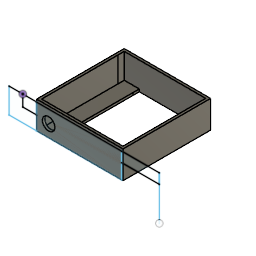
Battery_Body (Autodesk Fusion 360 design; units mm, degrees)
part number: 2026-04-07-23-47-39-558
Autodesk Fusion 360 part; units mm, degrees
sketch "Sketch1" plane through (0, 0, 0) normal (0, 1, 0) x (1, 0, 0)
  line L0 (0, 0) -> (11, 0)
  line L1 (11, 0) -> (11, 9)
  line L2 (11, 9) -> (0, 9)
  line L3 (0, 9) -> (0, 0)
  line L4 (11, 0) -> (79, 0)
  line L5 (79, 0) -> (79, 20)
  line L6 (79, 20) -> (11, 20)
  line L7 (11, 20) -> (11, 0)
  line L8 (11, 20) -> (-11, 20)
  line L9 (-11, 20) -> (-11, 0)
  line L10 (-11, 0) -> (0, 0)
  line L11 (79, 0) -> (109, 0)
  line L12 (109, 0) -> (109, 8)
  line L13 (109, 8) -> (79, 8)
  line L14 (109, 0) -> (109, 35)
  dimension "d2" = 9
  dimension "d3" = 30
  dimension "d4" = 8
  dimension "d5" = 35
  dimension "d6" = 68
  dimension "d7" = 20
  constraint coincident L0.start L3.end
  constraint horizontal L0
  constraint perpendicular L0 L1
  constraint perpendicular L1 L2
  constraint perpendicular L0 L3
  constraint perpendicular L1 L4
  constraint perpendicular L4 L5
  constraint perpendicular L5 L6
  constraint perpendicular L7 L8
  constraint perpendicular L6 L9
  constraint perpendicular L3 L10
  constraint perpendicular L5 L11
  constraint perpendicular L11 L12
  constraint coincident L5 L13.end
  constraint perpendicular L5 L13
  constraint perpendicular L11 L14
  measures "d2" distance of L0.end L1.end
  measures "d3" distance of L4.end L11.end
  measures "d4" distance of L11.end L12.end
  measures "d5" distance of L11.end L14.end
  measures "d6" distance of L5.end L6.end
  measures "d7" distance of L8.end L9.end
extrude "Extrude1" add sketch "Sketch1" along normal blind 65 contours L1 L4 L5 L6 L7
shell "Shell1" thickness 2 removed faces 1 at (33.6667, 21.6667, 0)
hole "Hole1" at (20.5975, 0, -10.3145) direction (0, 1, 0) diameter 10 depth 5 tip angle 180
sketch "Sketch2" plane through (0, 0, -18) normal (0, 0, 1) x (-1, 0, 0)
  line L0 (-13, -2) -> (-77, -2)
  line L1 (-77, -2) -> (-77, -63)
  line L2 (-77, -63) -> (-13, -63)
  line L3 (-13, -63) -> (-13, -2)
  line L4 (-13, -2) -> (-25, -2)
  line L5 (-25, -63) -> (-25, -2)
  line L6 (-77, -2) -> (-65, -2)
  line L7 (-65, -2) -> (-65, -63)
  line L8 (-77, -63) -> (-77, -2)
  line L9 (-25, -2) -> (-65, -2)
  line L10 (-65, -63) -> (-25, -63)
  dimension "d14" = 12
  constraint coincident L0.start L3.end
  constraint coincident L0 L4.end
  constraint coincident L2 L5.start
  constraint perpendicular L4 L5
  constraint coincident L0.end L1.start
  constraint perpendicular L1 L6
  constraint coincident L2 L7.end
  constraint perpendicular L2 L7
  constraint coincident L1.end L2.start
  measures "d14" distance of L0.end L6.end
extrude "Extrude2" cut sketch "Sketch2" against normal blind 5 contours L0 L2 L5 L7 L9 L10
extrude "Extrude3" add 1 faces at (34.3333, 64.3333, 0) along direction (0, 0, 1) blind 2
extrude "Extrude4" add 1 faces at (33.6667, 65, -5.3333) along direction (0, 1, 0) blind 5
sketch "Sketch3" plane through (0, 0, 2) normal (0, 0, 1) x (-1, 0, 0)
  line L0 (-13, -2) -> (-13, -63)
  line L1 (-13, -63) -> (-77, -63)
  line L2 (-77, -63) -> (-77, -2)
  line L3 (-77, -2) -> (-13, -2)
  line L4 (-11, 0) -> (-79, 0)
  line L5 (-79, 0) -> (-79, -70)
  line L6 (-79, -70) -> (-11, -70)
  line L7 (-11, -70) -> (-11, 0)
  line L8 (-77, -63) -> (-77, -68)
  line L9 (-77, -68) -> (-13, -68)
  line L10 (-13, -68) -> (-13, -63)
  constraint coincident L1.end L2.start
  constraint perpendicular L1 L8
  constraint perpendicular L8 L9
  constraint coincident L0.end L1.start
extrude "Extrude5" cut sketch "Sketch3" against normal blind 20 contours L1 L8 L9 L10
sketch "Sketch4" plane through (0, 0, -18) normal (0, 0, 1) x (-1, 0, 0)
  line L0 (-25, -2) -> (-25, -63)
  line L1 (-25, -63) -> (-65, -63)
  line L2 (-65, -63) -> (-65, -2)
  line L3 (-65, -2) -> (-77, -2)
  line L4 (-77, -2) -> (-77, -68)
  line L5 (-77, -68) -> (-13, -68)
  line L6 (-13, -68) -> (-13, -63)
  line L7 (-13, -63) -> (-13, -2)
  line L8 (-13, -2) -> (-25, -2)
  line L9 (-65, -63) -> (-65, -68)
  line L10 (-25, -68) -> (-25, -63)
  constraint coincident L1.end L2.start
  constraint coincident L5 L9.end
  constraint perpendicular L1 L9
  constraint coincident L5 L10.start
  constraint coincident L0.end L1.start
extrude "Extrude6" cut sketch "Sketch4" against normal blind 3 contours L1 L5 L9 L10
extrude "Extrude7" add 1 faces at (79, 46.6667, -12.6667) along direction (1, 0, 0) blind 1
extrude "Extrude8" cut 1 faces at (77, 44.3333, -4.6667) along direction (1, 0, 0) blind 1
extrude "Extrude9" cut 1 faces at (65, 44.3333, -19.3333) along direction (1, 0, 0) blind 1
